Autodesk Fusion 360 part; units mm, degrees
(part 3 of 4)
sketch "Esboço7" plane through (0, 0, 2) normal (0, 0, 1) x (-1, 0, 0)
  arc A0 (-89.8492, -89.6213) -> (-86.4551, -92.1669) centre (-86.8794, -89.1971) ccw
  arc A1 (-79.6669, -98.9551) -> (-86.4551, -92.1669) centre (-85.6066, -98.1066) ccw
  arc A2 (-79.6669, -98.9551) -> (-77.1213, -102.3492) centre (-76.6971, -99.3794) ccw
  arc A3 (-77.1213, -102.3492) -> (-73.7447, -102.4474) centre (-75, -87.5) ccw
  arc A4 (-46.7294, -108.889) -> (-73.7447, -102.4474) centre (-70.0264, -146.7235) ccw
  arc A5 (72.6915, -102.3213) -> (44.7852, -108.3244) centre (66.5604, -141.6847) ccw
  arc A6 (72.6915, -102.3213) -> (77.1213, -102.3492) centre (75, -87.5) ccw
  arc A7 (77.1213, -102.3492) -> (79.6669, -98.9551) centre (76.6971, -99.3794) ccw
  arc A8 (86.4551, -92.1669) -> (79.6669, -98.9551) centre (85.6066, -98.1066) ccw
  arc A9 (86.4551, -92.1669) -> (89.8492, -89.6213) centre (86.8794, -89.1971) ccw
  arc A10 (89.8492, -89.6213) -> (89.8492, -85.3787) centre (75, -87.5) ccw
  arc A11 (89.8492, -85.3787) -> (86.4551, -82.8331) centre (86.8794, -85.8029) ccw
  arc A12 (79.7798, -75.4623) -> (86.4551, -82.8331) centre (85.6066, -76.8934) ccw
  arc A13 (79.7798, -75.4623) -> (78.5519, -72.265) centre (76.8663, -74.7468) ccw
  arc A14 (60.7593, -50.7677) -> (78.5519, -72.265) centre (106.6436, -30.9026) ccw
  line L0 (60.7593, -50.7677) -> (50.5773, -27.2494)
  arc A15 (51.0282, 29.3922) -> (50.5773, -27.2494) centre (114.8154, 0.5617) ccw
  line L1 (51.0282, 29.3922) -> (60.9948, 51.443)
  arc A16 (78.5458, 72.2669) -> (60.9948, 51.443) centre (106.557, 30.8499) ccw
  arc A17 (78.5458, 72.2669) -> (79.7789, 75.4657) centre (76.8651, 74.7519) ccw
  arc A18 (86.4551, 82.8331) -> (79.7789, 75.4657) centre (85.6066, 76.8934) ccw
  arc A19 (86.4551, 82.8331) -> (89.8492, 85.3787) centre (86.8794, 85.8029) ccw
  arc A20 (89.8492, 85.3787) -> (89.8492, 89.6213) centre (75, 87.5) ccw
  arc A21 (89.8492, 89.6213) -> (86.4551, 92.1669) centre (86.8794, 89.1971) ccw
  arc A22 (79.6669, 98.9551) -> (86.4551, 92.1669) centre (85.6066, 98.1066) ccw
  arc A23 (79.6669, 98.9551) -> (77.1213, 102.3492) centre (76.6971, 99.3794) ccw
  arc A24 (77.1213, 102.3492) -> (72.8787, 102.3492) centre (75, 87.5) ccw
  arc A25 (72.8787, 102.3492) -> (70.3331, 98.9551) centre (73.3029, 99.3794) ccw
  arc A26 (62.5456, 92.3982) -> (70.3331, 98.9551) centre (64.3934, 98.1066) ccw
  arc A27 (62.5456, 92.3982) -> (59.6541, 91.8087) centre (61.6216, 89.544) ccw
  arc A28 (44.4663, 82.7551) -> (59.6541, 91.8087) centre (26.8616, 129.5533) ccw
  arc A29 (-59.6538, 91.7779) -> (-44.9685, 82.7086) centre (-26.4329, 129.146) ccw
  arc A30 (-59.6538, 91.7779) -> (-62.5625, 92.3928) centre (-61.6471, 89.5359) ccw
  arc A31 (-70.3331, 98.9551) -> (-62.5625, 92.3928) centre (-64.3934, 98.1066) ccw
  arc A32 (-70.3331, 98.9551) -> (-72.8787, 102.3492) centre (-73.3029, 99.3794) ccw
  arc A33 (-72.8787, 102.3492) -> (-77.1213, 102.3492) centre (-75, 87.5) ccw
  arc A34 (-77.1213, 102.3492) -> (-79.6669, 98.9551) centre (-76.6971, 99.3794) ccw
  arc A35 (-86.4551, 92.1669) -> (-79.6669, 98.9551) centre (-85.6066, 98.1066) ccw
  arc A36 (-86.4551, 92.1669) -> (-89.8492, 89.6213) centre (-86.8794, 89.1971) ccw
  arc A37 (-89.8492, 89.6213) -> (-89.8492, 85.3787) centre (-75, 87.5) ccw
  arc A38 (-89.8492, 85.3787) -> (-86.4551, 82.8331) centre (-86.8794, 85.8029) ccw
  arc A39 (-79.7789, 75.4657) -> (-86.4551, 82.8331) centre (-85.6066, 76.8934) ccw
  arc A40 (-79.7789, 75.4657) -> (-78.5458, 72.2669) centre (-76.8651, 74.7519) ccw
  arc A41 (-60.9948, 51.443) -> (-78.5458, 72.2669) centre (-106.557, 30.8499) ccw
  line L2 (-60.9948, 51.443) -> (-51.0282, 29.3922)
  arc A42 (-50.5773, -27.2494) -> (-51.0282, 29.3922) centre (-114.8154, 0.5617) ccw
  line L3 (-50.5773, -27.2494) -> (-60.7593, -50.7677)
  arc A43 (-78.5519, -72.265) -> (-60.7593, -50.7677) centre (-106.6436, -30.9026) ccw
  arc A44 (-78.5519, -72.265) -> (-79.7798, -75.4623) centre (-76.8663, -74.7468) ccw
  arc A45 (-86.4551, -82.8331) -> (-79.7798, -75.4623) centre (-85.6066, -76.8934) ccw
  arc A46 (-86.4551, -82.8331) -> (-89.8492, -85.3787) centre (-86.8794, -85.8029) ccw
  arc A47 (-89.8492, -85.3787) -> (-89.8492, -89.6213) centre (-75, -87.5) ccw
  circle A48 centre (72.5, -95.6021) radius 1.5
  circle A49 centre (-83, -87.5005) radius 1.5
  circle A50 centre (-75.0002, 95.5) radius 1.5
  circle A51 centre (-67, 87.5002) radius 1.5
  circle A52 centre (83, 87.5) radius 1.5
  circle A53 centre (75, 79.5) radius 1.5
  circle A54 centre (-75, 87.5) radius 3
  circle A55 centre (-74.9995, -95.5) radius 1.5
  circle A56 centre (-75.0005, -79.5) radius 1.5
  circle A57 centre (64.5, -87.6021) radius 1.5
  circle A58 centre (80.5, -87.6021) radius 1.5
  circle A59 centre (-75, -87.5) radius 3
  circle A60 centre (-83, 87.4998) radius 1.5
  circle A61 centre (75, 95.5) radius 1.5
  circle A62 centre (75, 87.5) radius 3
  circle A63 centre (67, 87.5) radius 1.5
  circle A64 centre (-74.9998, 79.5) radius 1.5
  circle A65 centre (-67, -87.4995) radius 1.5
  circle A66 centre (75, -87.5) radius 3
  circle A67 centre (72.5, -79.6021) radius 1.5
  circle A68 centre (40.65, 50) radius 2.15
  arc A69 (-57.5607, 76.943) -> (-64.8173, 70.6939) centre (-60.2496, 72.7276) ccw
  line L4 (-57.5607, 76.943) -> (-49.4611, 71.7764)
  arc A70 (-47.15, 67.561) -> (-49.4611, 71.7764) centre (-52.15, 67.561) ccw
  line L5 (-47.15, 67.561) -> (-47.15, 42.4858)
  arc A71 (-47.4521, 41.7697) -> (-47.15, 42.4858) centre (-48.15, 42.4858) ccw
  line L6 (-47.4521, 41.7697) -> (-49.5538, 39.7214)
  arc A72 (-51.1653, 40.0309) -> (-49.5538, 39.7214) centre (-50.2517, 40.4376) ccw
  line L7 (-51.1653, 40.0309) -> (-64.8173, 70.6939)
  circle A73 centre (-40.65, 50) radius 2.15
  circle A74 centre (40.65, 60) radius 2.15
  line L8 (47.15, 42.4858) -> (47.15, 67.561)
  arc A75 (49.4611, 71.7764) -> (47.15, 67.561) centre (52.15, 67.561) ccw
  line L9 (49.4611, 71.7764) -> (57.5607, 76.943)
  arc A76 (64.8173, 70.6939) -> (57.5607, 76.943) centre (60.2496, 72.7276) ccw
  line L10 (64.8173, 70.6939) -> (51.1653, 40.0309)
  arc A77 (49.5538, 39.7214) -> (51.1653, 40.0309) centre (50.2517, 40.4376) ccw
  line L11 (49.5538, 39.7214) -> (47.4521, 41.7697)
  arc A78 (47.15, 42.4858) -> (47.4521, 41.7697) centre (48.15, 42.4858) ccw
  circle A79 centre (-40.65, 60) radius 2.15
  arc A80 (-10.473, -56.6595) -> (-14.3032, -58.4456) centre (-10.473, -61.6595) ccw
  line L12 (-10.473, -56.6595) -> (-7, -56.6595)
  arc A81 (-5, -58.6595) -> (-7, -56.6595) centre (-7, -58.6595) ccw
  line L13 (-5, -58.6595) -> (-5, -97.464)
  arc A82 (-9.1318, -102.3881) -> (-5, -97.464) centre (-10, -97.464) ccw
  line L14 (-9.1318, -102.3881) -> (-26.9725, -105.5339)
  arc A83 (-32.7648, -101.4781) -> (-26.9725, -105.5339) centre (-27.8408, -100.6098) ccw
  line L15 (-32.7648, -101.4781) -> (-35.4243, -86.3954)
  arc A84 (-34.3305, -82.3132) -> (-35.4243, -86.3954) centre (-30.5003, -85.5271) ccw
  line L16 (-34.3305, -82.3132) -> (-14.3032, -58.4456)
  arc A85 (-40.9054, 16.7074) -> (-37.3489, 15.6517) centre (-38.8619, 17.0732) ccw
  line L17 (-40.9054, 16.7074) -> (-46.7322, 29.5993)
  arc A86 (-44.339, 36.0244) -> (-46.7322, 29.5993) centre (-42.0339, 31.5075) ccw
  arc A87 (-44.339, 36.0244) -> (-34.6129, 45.4956) centre (-56.2565, 57.9923) ccw
  arc A88 (-28.1234, 47.5076) -> (-34.6129, 45.4956) centre (-30.28, 42.9921) ccw
  line L18 (-28.1234, 47.5076) -> (-14.9942, 41.2515)
  arc A89 (-14.46, 38.0146) -> (-14.9942, 41.2515) centre (-15.8549, 39.4469) ccw
  line L19 (-14.46, 38.0146) -> (-37.3489, 15.6517)
  line L20 (5, -97.464) -> (5, -58.6595)
  arc A90 (7, -56.6595) -> (5, -58.6595) centre (7, -58.6595) ccw
  line L21 (7, -56.6595) -> (10.473, -56.6595)
  arc A91 (14.3032, -58.4456) -> (10.473, -56.6595) centre (10.473, -61.6595) ccw
  line L22 (14.3032, -58.4456) -> (34.3305, -82.3132)
  arc A92 (35.4243, -86.3954) -> (34.3305, -82.3132) centre (30.5003, -85.5271) ccw
  line L23 (35.4243, -86.3954) -> (32.7648, -101.4781)
  arc A93 (26.9725, -105.5339) -> (32.7648, -101.4781) centre (27.8408, -100.6098) ccw
  line L24 (26.9725, -105.5339) -> (9.1318, -102.3881)
  arc A94 (5, -97.464) -> (9.1318, -102.3881) centre (10, -97.464) ccw
  arc A95 (-61.9967, -63.6938) -> (-55.4143, -68.0759) centre (-58.3695, -65.3802) ccw
  line L25 (-61.9967, -63.6938) -> (-41.8922, -17.2564)
  arc A96 (-36.246, -16.5772) -> (-41.8922, -17.2564) centre (-38.8636, -18.6251) ccw
  line L26 (-36.246, -16.5772) -> (-23.6374, -29.1331)
  arc A97 (-23.5625, -33.2372) -> (-23.6374, -29.1331) centre (-25.7596, -31.2246) ccw
  line L27 (-23.5625, -33.2372) -> (-55.4143, -68.0759)
  arc A98 (38.1376, -9.2791) -> (38.7256, -7.6527) centre (36.7356, -7.8528) ccw
  line L28 (38.1376, -9.2791) -> (27.9736, -19.2699)
  arc A99 (24.5716, -17.8424) -> (27.9736, -19.2699) centre (26.5716, -17.8436) ccw
  line L29 (24.5716, -17.8424) -> (24.5916, 17.8264)
  arc A100 (27.9955, 19.2498) -> (24.5916, 17.8264) centre (26.5916, 17.8253) ccw
  line L30 (27.9955, 19.2498) -> (38.1463, 9.2454)
  arc A101 (38.7321, 7.6192) -> (38.1463, 9.2454) centre (36.7424, 7.821) ccw
  arc A102 (38.7321, 7.6192) -> (38.7256, -7.6527) centre (114.3432, -0.0492) ccw
  arc A103 (9.266, 38.142) -> (7.6383, 38.7303) centre (7.8393, 36.7404) ccw
  line L31 (9.266, 38.142) -> (19.2664, 27.9622)
  arc A104 (17.8415, 24.5606) -> (19.2664, 27.9622) centre (17.8397, 26.5606) ccw
  line L32 (17.8415, 24.5606) -> (-17.871, 24.5283)
  arc A105 (-19.3052, 27.9241) -> (-17.871, 24.5283) centre (-17.8728, 26.5283) ccw
  line L33 (-19.3052, 27.9241) -> (-9.3455, 38.1438)
  arc A106 (-7.7103, 38.7376) -> (-9.3455, 38.1438) centre (-7.9132, 36.7479) ccw
  arc A107 (-7.7103, 38.7376) -> (7.6383, 38.7303) centre (0, 114.3455) ccw
  line L34 (41.7895, -17.0192) -> (61.9965, -63.6935)
  arc A108 (55.3948, -68.0303) -> (61.9965, -63.6935) centre (58.3475, -65.3318) ccw
  line L35 (55.3948, -68.0303) -> (23.5953, -33.2362)
  arc A109 (23.7067, -29.0729) -> (23.5953, -33.2362) centre (25.8097, -31.2123) ccw
  line L36 (23.7067, -29.0729) -> (36.9334, -16.0716)
  arc A110 (41.7895, -17.0192) -> (36.9334, -16.0716) centre (39.0364, -18.2111) ccw
  arc A111 (37.4337, 15.5639) -> (40.6601, 16.1647) centre (38.8376, 16.9884) ccw
  line L37 (37.4337, 15.5639) -> (14.6425, 38.0264)
  arc A112 (15.1963, 41.2612) -> (14.6425, 38.0264) centre (16.0464, 39.4508) ccw
  line L38 (15.1963, 41.2612) -> (28.3187, 47.4234)
  arc A113 (34.7856, 45.3775) -> (28.3187, 47.4234) centre (30.444, 42.8975) ccw
  arc A114 (34.7856, 45.3775) -> (44.4886, 35.8486) centre (56.4937, 57.7776) ccw
  arc A115 (46.6438, 29.4035) -> (44.4886, 35.8486) centre (42.0875, 31.4628) ccw
  line L39 (46.6438, 29.4035) -> (40.6601, 16.1647)
  line L40 (19.3052, -27.9241) -> (9.3455, -38.1438)
  arc A116 (7.7103, -38.7376) -> (9.3455, -38.1438) centre (7.9132, -36.7479) ccw
  arc A117 (7.7103, -38.7376) -> (-7.6383, -38.7303) centre (0, -114.3455) ccw
  arc A118 (-9.266, -38.142) -> (-7.6383, -38.7303) centre (-7.8393, -36.7404) ccw
  line L41 (-9.266, -38.142) -> (-19.2664, -27.9622)
  arc A119 (-17.8415, -24.5606) -> (-19.2664, -27.9622) centre (-17.8397, -26.5606) ccw
  line L42 (-17.8415, -24.5606) -> (17.871, -24.5283)
  arc A120 (19.3052, -27.9241) -> (17.871, -24.5283) centre (17.8728, -26.5283) ccw
  arc A121 (-38.7303, -7.6383) -> (-38.142, -9.266) centre (-36.7404, -7.8393) ccw
  arc A122 (-38.7303, -7.6383) -> (-38.7376, 7.7103) centre (-114.3455, 0) ccw
  arc A123 (-38.1438, 9.3455) -> (-38.7376, 7.7103) centre (-36.7479, 7.9132) ccw
  line L43 (-38.1438, 9.3455) -> (-27.9241, 19.3052)
  arc A124 (-24.5283, 17.871) -> (-27.9241, 19.3052) centre (-26.5283, 17.8728) ccw
  line L44 (-24.5283, 17.871) -> (-24.5606, -17.8415)
  arc A125 (-27.9622, -19.2664) -> (-24.5607, -17.8415) centre (-26.5606, -17.8397) ccw
  line L45 (-27.9622, -19.2664) -> (-38.142, -9.266)
  circle A126 centre (-10.25, -46.6) radius 1.5
  line L46 (8, -42.5) -> (8, -50.7)
  line L47 (8, -50.7) -> (-8, -50.7)
  line L48 (-8, -50.7) -> (-8, -42.5)
  line L49 (-8, -42.5) -> (8, -42.5)
  circle A127 centre (10.25, -46.6) radius 1.5
  circle A128 centre (-50, 0) radius 2.15
  arc A129 (-50.5733, 28.3637) -> (-50.5773, -27.2494) centre (35.4576, 0.5509) ccw
  line L50 (0, 0) -> (0, -46.9846) construction
  circle A130 centre (50, 0) radius 2.15
  arc A131 (50.5773, -27.2494) -> (50.5733, 28.3637) centre (-35.4576, 0.5509) ccw
  line L51 (35.9657, 79.8952) -> (2.1827, 93.0889)
  arc A132 (2.1827, 93.0889) -> (-2.1423, 93.1045) centre (0, 87.5) ccw
  line L52 (0, 81.5) -> (15.6612, 75.3836)
  line L53 (-16.4256, 75.2214) -> (0, 81.5)
  line L54 (-2.1423, 93.1045) -> (-36.9275, 79.8081)
  arc A133 (6.7322, 8.1464) -> (6.3787, 9) centre (6.3787, 8.5) ccw
  line L55 (6.7322, 8.1464) -> (0.7071, 2.1213)
  arc A134 (-0.7071, 2.1213) -> (0.7071, 2.1213) centre (0, 2.8284) ccw
  line L56 (-0.7071, 2.1213) -> (-6.7322, 8.1464)
  arc A135 (-6.3787, 9) -> (-6.7322, 8.1464) centre (-6.3787, 8.5) ccw
  line L57 (-6.3787, 9) -> (6.3787, 9)
  arc A136 (-8.1464, 6.7322) -> (-9, 6.3787) centre (-8.5, 6.3787) ccw
  line L58 (-8.1464, 6.7322) -> (-2.1213, 0.7071)
  arc A137 (-2.1213, -0.7071) -> (-2.1213, 0.7071) centre (-2.8284, 0) ccw
  line L59 (-2.1213, -0.7071) -> (-8.1464, -6.7322)
  arc A138 (-9, -6.3787) -> (-8.1464, -6.7322) centre (-8.5, -6.3787) ccw
  line L60 (-9, -6.3787) -> (-9, 6.3787)
  arc A139 (-6.7322, -8.1464) -> (-6.3787, -9) centre (-6.3787, -8.5) ccw
  line L61 (-6.7322, -8.1464) -> (-0.7071, -2.1213)
  arc A140 (0.7071, -2.1213) -> (-0.7071, -2.1213) centre (0, -2.8284) ccw
  line L62 (0.7071, -2.1213) -> (6.7322, -8.1464)
  arc A141 (6.3787, -9) -> (6.7322, -8.1464) centre (6.3787, -8.5) ccw
  line L63 (6.3787, -9) -> (-6.3787, -9)
  line L64 (8.1464, -6.7322) -> (2.1213, -0.7071)
  arc A142 (2.1213, 0.7071) -> (2.1213, -0.7071) centre (2.8284, 0) ccw
  line L65 (2.1213, 0.7071) -> (8.1464, 6.7322)
  arc A143 (9, 6.3787) -> (8.1464, 6.7322) centre (8.5, 6.3787) ccw
  line L66 (9, 6.3787) -> (9, -6.3787)
  arc A144 (8.1464, -6.7322) -> (9, -6.3787) centre (8.5, -6.3787) ccw
  circle A145 centre (0, 87.5) radius 2.15
  arc A146 (26.2105, 50.915) -> (27.5676, 55.0697) centre (24.9353, 53.6305) ccw
  line L67 (26.2105, 50.915) -> (10.6059, 43.5872)
  arc A147 (9.3307, 43.3027) -> (10.6059, 43.5872) centre (9.3307, 46.3027) ccw
  line L68 (9.3307, 43.3027) -> (-9.3218, 43.3027)
  arc A148 (-10.6123, 43.5944) -> (-9.3218, 43.3027) centre (-9.3218, 46.3027) ccw
  line L69 (-10.6123, 43.5944) -> (-26.8632, 51.3381)
  arc A149 (-28.1945, 55.5044) -> (-26.8632, 51.3381) centre (-25.5727, 54.0463) ccw
  line L70 (-28.1945, 55.5044) -> (-17.9762, 73.8773)
  arc A150 (-16.4256, 75.2214) -> (-17.9762, 73.8773) centre (-15.3544, 72.4192) ccw
  arc A151 (17.2021, 74.0283) -> (15.6612, 75.3836) centre (14.5698, 72.5892) ccw
  line L71 (17.2021, 74.0283) -> (27.5676, 55.0697)
  arc A152 (-46.7294, -108.889) -> (-25.7561, -114.8285) centre (-25.7561, -74.8285) ccw
  line L72 (-25.7561, -114.8285) -> (22.9214, -114.8285)
  arc A153 (22.9214, -114.8285) -> (44.7852, -108.3244) centre (22.9214, -74.8285) ccw
  circle A154 centre (-10, 10) radius 3
  circle A155 centre (10, -10) radius 3
  circle A156 centre (-10, -10) radius 3
  circle A157 centre (10, 10) radius 3
  arc A158 (35.9657, 79.8952) -> (44.4663, 82.7551) centre (-0.31, 201.7835) ccw
  arc A159 (-44.9685, 82.7086) -> (-36.9275, 79.8081) centre (2.2046, 200.8918) ccw
  point P0 (-72.5, 87.3979)
  point P1 (-72.5, -87.6021)
  point P2 (72.5, 87.3979)
  point P3 (72.5, -87.6021)
  point P4 (-72.5, 87.3979)
  point P5 (-72.5, -87.6021)
  point P6 (72.5, 87.3979)
  point P7 (72.5, -87.6021)
  point P8 (-72.5, 87.3979)
  point P9 (-72.5, -87.6021)
  point P10 (72.5, 87.3979)
  point P11 (72.5, -87.6021)
  point P12 (-72.5, 87.3979)
  point P13 (-72.5, -87.6021)
  point P14 (72.5, 87.3979)
  point P15 (72.5, -87.6021)
  point P16 (-72.5, 87.3979)
  point P17 (-72.5, -87.6021)
  point P18 (72.5, 87.3979)
  point P19 (72.5, -87.6021)
  point P20 (72.5, -87.6021)
  point P21 (72.5, -87.6021)
  point P22 (72.5, -87.6021)
  point P23 (72.5, -87.6021)
  dimension "d142" = 4.3
  dimension "d143" = 50
  dimension "d144" = 90.4149
  constraint coincident A42.start L3.start
  constraint coincident L50.start origin
  constraint perpendicular L49 L50
  constraint symmetric A128 L50 A130
  constraint symmetric A42.start L50 L0.end
  constraint symmetric A129.start L50 A131.end
  constraint symmetric A129 L50 A131
  constraint coincident A15 A131.end
  measures "d142" diameter of A128
  measures "d143" distance of L50.start A128.centre
  measures "d144" radius of A129
extrude "Extrusão9" add sketch "Esboço7" against normal blind 4 contours A42 A129 | A15 A131
fillet "Arredondamento3" radius 15 4 edges at (50.5733, -28.3637, 0) (50.5773, 27.2494, 0) (-50.5733, -28.3637, 0) (-50.5773, 27.2494, 0)
sketch "Esboço8" plane through (0, 0, 2) normal (0, 0, 1) x (-1, 0, 0)
  circle A0 centre (-50, 0) radius 2.15
  circle A1 centre (50, 0) radius 2.15
  arc A2 (-89.8492, -89.6213) -> (-86.4551, -92.1669) centre (-86.8794, -89.1971) ccw
  arc A3 (-79.6669, -98.9551) -> (-86.4551, -92.1669) centre (-85.6066, -98.1066) ccw
  arc A4 (-79.6669, -98.9551) -> (-77.1213, -102.3492) centre (-76.6971, -99.3794) ccw
  arc A5 (-77.1213, -102.3492) -> (-73.7447, -102.4474) centre (-75, -87.5) ccw
  arc A6 (-46.7294, -108.889) -> (-73.7447, -102.4474) centre (-70.0264, -146.7235) ccw
  arc A7 (72.6915, -102.3213) -> (44.7852, -108.3244) centre (66.5604, -141.6847) ccw
  arc A8 (72.6915, -102.3213) -> (77.1213, -102.3492) centre (75, -87.5) ccw
  arc A9 (77.1213, -102.3492) -> (79.6669, -98.9551) centre (76.6971, -99.3794) ccw
  arc A10 (86.4551, -92.1669) -> (79.6669, -98.9551) centre (85.6066, -98.1066) ccw
  arc A11 (86.4551, -92.1669) -> (89.8492, -89.6213) centre (86.8794, -89.1971) ccw
  arc A12 (89.8492, -89.6213) -> (89.8492, -85.3787) centre (75, -87.5) ccw
  arc A13 (89.8492, -85.3787) -> (86.4551, -82.8331) centre (86.8794, -85.8029) ccw
  arc A14 (79.7798, -75.4623) -> (86.4551, -82.8331) centre (85.6066, -76.8934) ccw
  arc A15 (79.7798, -75.4623) -> (78.5519, -72.265) centre (76.8663, -74.7468) ccw
  arc A16 (60.7593, -50.7677) -> (78.5519, -72.265) centre (106.6436, -30.9026) ccw
  line L0 (60.7593, -50.7677) -> (52.7268, -32.2145)
  arc A17 (51.9852, -22.4406) -> (52.7268, -32.2145) centre (66.4922, -26.2549) ccw
  arc A18 (51.9852, -22.4406) -> (52.0095, 23.4499) centre (-35.4576, 0.5509) ccw
  arc A19 (52.8518, 33.4268) -> (52.0095, 23.4499) centre (66.5205, 27.2489) ccw
  line L1 (52.8518, 33.4268) -> (60.9948, 51.443)
  arc A20 (78.5458, 72.2669) -> (60.9948, 51.443) centre (106.557, 30.8499) ccw
  arc A21 (78.5458, 72.2669) -> (79.7789, 75.4657) centre (76.8651, 74.7519) ccw
  arc A22 (86.4551, 82.8331) -> (79.7789, 75.4657) centre (85.6066, 76.8934) ccw
  arc A23 (86.4551, 82.8331) -> (89.8492, 85.3787) centre (86.8794, 85.8029) ccw
  arc A24 (89.8492, 85.3787) -> (89.8492, 89.6213) centre (75, 87.5) ccw
  arc A25 (89.8492, 89.6213) -> (86.4551, 92.1669) centre (86.8794, 89.1971) ccw
  arc A26 (79.6669, 98.9551) -> (86.4551, 92.1669) centre (85.6066, 98.1066) ccw
  arc A27 (79.6669, 98.9551) -> (77.1213, 102.3492) centre (76.6971, 99.3794) ccw
  arc A28 (77.1213, 102.3492) -> (72.8787, 102.3492) centre (75, 87.5) ccw
  arc A29 (72.8787, 102.3492) -> (70.3331, 98.9551) centre (73.3029, 99.3794) ccw
  arc A30 (62.5456, 92.3982) -> (70.3331, 98.9551) centre (64.3934, 98.1066) ccw
  arc A31 (62.5456, 92.3982) -> (59.6541, 91.8087) centre (61.6216, 89.544) ccw
  arc A32 (44.4663, 82.7551) -> (59.6541, 91.8087) centre (26.8616, 129.5533) ccw
  arc A33 (-59.6538, 91.7779) -> (-44.9685, 82.7086) centre (-26.4329, 129.146) ccw
  arc A34 (-59.6538, 91.7779) -> (-62.5625, 92.3928) centre (-61.6471, 89.5359) ccw
  arc A35 (-70.3331, 98.9551) -> (-62.5625, 92.3928) centre (-64.3934, 98.1066) ccw
  arc A36 (-70.3331, 98.9551) -> (-72.8787, 102.3492) centre (-73.3029, 99.3794) ccw
  arc A37 (-72.8787, 102.3492) -> (-77.1213, 102.3492) centre (-75, 87.5) ccw
  arc A38 (-77.1213, 102.3492) -> (-79.6669, 98.9551) centre (-76.6971, 99.3794) ccw
  arc A39 (-86.4551, 92.1669) -> (-79.6669, 98.9551) centre (-85.6066, 98.1066) ccw
  arc A40 (-86.4551, 92.1669) -> (-89.8492, 89.6213) centre (-86.8794, 89.1971) ccw
  arc A41 (-89.8492, 89.6213) -> (-89.8492, 85.3787) centre (-75, 87.5) ccw
  arc A42 (-89.8492, 85.3787) -> (-86.4551, 82.8331) centre (-86.8794, 85.8029) ccw
  arc A43 (-79.7789, 75.4657) -> (-86.4551, 82.8331) centre (-85.6066, 76.8934) ccw
  arc A44 (-79.7789, 75.4657) -> (-78.5458, 72.2669) centre (-76.8651, 74.7519) ccw
  arc A45 (-60.9948, 51.443) -> (-78.5458, 72.2669) centre (-106.557, 30.8499) ccw
  line L2 (-60.9948, 51.443) -> (-52.8518, 33.4268)
  arc A46 (-52.0095, 23.4499) -> (-52.8518, 33.4268) centre (-66.5205, 27.2489) ccw
  arc A47 (-52.0095, 23.4499) -> (-51.9852, -22.4406) centre (35.4576, 0.5509) ccw
  arc A48 (-52.7268, -32.2145) -> (-51.9852, -22.4406) centre (-66.4922, -26.2549) ccw
  line L3 (-52.7268, -32.2145) -> (-60.7593, -50.7677)
  arc A49 (-78.5519, -72.265) -> (-60.7593, -50.7677) centre (-106.6436, -30.9026) ccw
  arc A50 (-78.5519, -72.265) -> (-79.7798, -75.4623) centre (-76.8663, -74.7468) ccw
  arc A51 (-86.4551, -82.8331) -> (-79.7798, -75.4623) centre (-85.6066, -76.8934) ccw
  arc A52 (-86.4551, -82.8331) -> (-89.8492, -85.3787) centre (-86.8794, -85.8029) ccw
  arc A53 (-89.8492, -85.3787) -> (-89.8492, -89.6213) centre (-75, -87.5) ccw
  circle A54 centre (72.5, -95.6021) radius 1.5
  circle A55 centre (-83, -87.5005) radius 1.5
  circle A56 centre (-75.0002, 95.5) radius 1.5
  circle A57 centre (-67, 87.5002) radius 1.5
  circle A58 centre (83, 87.5) radius 1.5
  circle A59 centre (75, 79.5) radius 1.5
  circle A60 centre (-75, 87.5) radius 3
  circle A61 centre (-74.9995, -95.5) radius 1.5
  circle A62 centre (-75.0005, -79.5) radius 1.5
  circle A63 centre (64.5, -87.6021) radius 1.5
  circle A64 centre (80.5, -87.6021) radius 1.5
  circle A65 centre (-75, -87.5) radius 3
  circle A66 centre (-83, 87.4998) radius 1.5
  circle A67 centre (75, 95.5) radius 1.5
  circle A68 centre (75, 87.5) radius 3
  circle A69 centre (67, 87.5) radius 1.5
  circle A70 centre (-74.9998, 79.5) radius 1.5
  circle A71 centre (-67, -87.4995) radius 1.5
  circle A72 centre (75, -87.5) radius 3
  circle A73 centre (72.5, -79.6021) radius 1.5
  circle A74 centre (40.65, 50) radius 2.15
  arc A75 (-57.5607, 76.943) -> (-64.8173, 70.6939) centre (-60.2496, 72.7276) ccw
  line L4 (-57.5607, 76.943) -> (-49.4611, 71.7764)
  arc A76 (-47.15, 67.561) -> (-49.4611, 71.7764) centre (-52.15, 67.561) ccw
  line L5 (-47.15, 67.561) -> (-47.15, 42.4858)
  arc A77 (-47.4521, 41.7697) -> (-47.15, 42.4858) centre (-48.15, 42.4858) ccw
  line L6 (-47.4521, 41.7697) -> (-49.5538, 39.7214)
  arc A78 (-51.1653, 40.0309) -> (-49.5538, 39.7214) centre (-50.2517, 40.4376) ccw
  line L7 (-51.1653, 40.0309) -> (-64.8173, 70.6939)
  circle A79 centre (-40.65, 50) radius 2.15
  circle A80 centre (40.65, 60) radius 2.15
  line L8 (47.15, 42.4858) -> (47.15, 67.561)
  arc A81 (49.4611, 71.7764) -> (47.15, 67.561) centre (52.15, 67.561) ccw
  line L9 (49.4611, 71.7764) -> (57.5607, 76.943)
  arc A82 (64.8173, 70.6939) -> (57.5607, 76.943) centre (60.2496, 72.7276) ccw
  line L10 (64.8173, 70.6939) -> (51.1653, 40.0309)
  arc A83 (49.5538, 39.7214) -> (51.1653, 40.0309) centre (50.2517, 40.4376) ccw
  line L11 (49.5538, 39.7214) -> (47.4521, 41.7697)
  arc A84 (47.15, 42.4858) -> (47.4521, 41.7697) centre (48.15, 42.4858) ccw
  circle A85 centre (-40.65, 60) radius 2.15
  arc A86 (-10.473, -56.6595) -> (-14.3032, -58.4456) centre (-10.473, -61.6595) ccw
  line L12 (-10.473, -56.6595) -> (-7, -56.6595)
  arc A87 (-5, -58.6595) -> (-7, -56.6595) centre (-7, -58.6595) ccw
  line L13 (-5, -58.6595) -> (-5, -97.464)
  arc A88 (-9.1318, -102.3881) -> (-5, -97.464) centre (-10, -97.464) ccw
  line L14 (-9.1318, -102.3881) -> (-26.9725, -105.5339)
  arc A89 (-32.7648, -101.4781) -> (-26.9725, -105.5339) centre (-27.8408, -100.6098) ccw
  line L15 (-32.7648, -101.4781) -> (-35.4243, -86.3954)
  arc A90 (-34.3305, -82.3132) -> (-35.4243, -86.3954) centre (-30.5003, -85.5271) ccw
  line L16 (-34.3305, -82.3132) -> (-14.3032, -58.4456)
  arc A91 (-40.9054, 16.7074) -> (-37.3489, 15.6517) centre (-38.8619, 17.0732) ccw
  line L17 (-40.9054, 16.7074) -> (-46.7322, 29.5993)
  arc A92 (-44.339, 36.0244) -> (-46.7322, 29.5993) centre (-42.0339, 31.5075) ccw
  arc A93 (-44.339, 36.0244) -> (-34.6129, 45.4956) centre (-56.2565, 57.9923) ccw
  arc A94 (-28.1234, 47.5076) -> (-34.6129, 45.4956) centre (-30.28, 42.9921) ccw
  line L18 (-28.1234, 47.5076) -> (-14.9942, 41.2515)
  arc A95 (-14.46, 38.0146) -> (-14.9942, 41.2515) centre (-15.8549, 39.4469) ccw
  line L19 (-14.46, 38.0146) -> (-37.3489, 15.6517)
  line L20 (5, -97.464) -> (5, -58.6595)
  arc A96 (7, -56.6595) -> (5, -58.6595) centre (7, -58.6595) ccw
  line L21 (7, -56.6595) -> (10.473, -56.6595)
  arc A97 (14.3032, -58.4456) -> (10.473, -56.6595) centre (10.473, -61.6595) ccw
  line L22 (14.3032, -58.4456) -> (34.3305, -82.3132)
  arc A98 (35.4243, -86.3954) -> (34.3305, -82.3132) centre (30.5003, -85.5271) ccw
  line L23 (35.4243, -86.3954) -> (32.7648, -101.4781)
  arc A99 (26.9725, -105.5339) -> (32.7648, -101.4781) centre (27.8408, -100.6098) ccw
  line L24 (26.9725, -105.5339) -> (9.1318, -102.3881)
  arc A100 (5, -97.464) -> (9.1318, -102.3881) centre (10, -97.464) ccw
  arc A101 (-61.9967, -63.6938) -> (-55.4143, -68.0759) centre (-58.3695, -65.3802) ccw
  line L25 (-61.9967, -63.6938) -> (-41.8922, -17.2564)
  arc A102 (-36.246, -16.5772) -> (-41.8922, -17.2564) centre (-38.8636, -18.6251) ccw
  line L26 (-36.246, -16.5772) -> (-23.6374, -29.1331)
  arc A103 (-23.5625, -33.2372) -> (-23.6374, -29.1331) centre (-25.7596, -31.2246) ccw
  line L27 (-23.5625, -33.2372) -> (-55.4143, -68.0759)
  arc A104 (38.1376, -9.2791) -> (38.7256, -7.6527) centre (36.7356, -7.8528) ccw
  line L28 (38.1376, -9.2791) -> (27.9736, -19.2699)
  arc A105 (24.5716, -17.8424) -> (27.9736, -19.2699) centre (26.5716, -17.8436) ccw
  line L29 (24.5716, -17.8424) -> (24.5916, 17.8264)
  arc A106 (27.9955, 19.2498) -> (24.5916, 17.8264) centre (26.5916, 17.8253) ccw
  line L30 (27.9955, 19.2498) -> (38.1463, 9.2454)
  arc A107 (38.7321, 7.6192) -> (38.1463, 9.2454) centre (36.7424, 7.821) ccw
  arc A108 (38.7321, 7.6192) -> (38.7256, -7.6527) centre (114.3432, -0.0492) ccw
  arc A109 (9.266, 38.142) -> (7.6383, 38.7303) centre (7.8393, 36.7404) ccw
  line L31 (9.266, 38.142) -> (19.2664, 27.9622)
  arc A110 (17.8415, 24.5606) -> (19.2664, 27.9622) centre (17.8397, 26.5606) ccw
  line L32 (17.8415, 24.5606) -> (-17.871, 24.5283)
  arc A111 (-19.3052, 27.9241) -> (-17.871, 24.5283) centre (-17.8728, 26.5283) ccw
  line L33 (-19.3052, 27.9241) -> (-9.3455, 38.1438)
  arc A112 (-7.7103, 38.7376) -> (-9.3455, 38.1438) centre (-7.9132, 36.7479) ccw
  arc A113 (-7.7103, 38.7376) -> (7.6383, 38.7303) centre (0, 114.3455) ccw
  line L34 (41.7895, -17.0192) -> (61.9965, -63.6935)
  arc A114 (55.3948, -68.0303) -> (61.9965, -63.6935) centre (58.3475, -65.3318) ccw
  line L35 (55.3948, -68.0303) -> (23.5953, -33.2362)
  arc A115 (23.7067, -29.0729) -> (23.5953, -33.2362) centre (25.8097, -31.2123) ccw
  line L36 (23.7067, -29.0729) -> (36.9334, -16.0716)
  arc A116 (41.7895, -17.0192) -> (36.9334, -16.0716) centre (39.0364, -18.2111) ccw
  arc A117 (37.4337, 15.5639) -> (40.6601, 16.1647) centre (38.8376, 16.9884) ccw
  line L37 (37.4337, 15.5639) -> (14.6425, 38.0264)
  arc A118 (15.1963, 41.2612) -> (14.6425, 38.0264) centre (16.0464, 39.4508) ccw
  line L38 (15.1963, 41.2612) -> (28.3187, 47.4234)
  arc A119 (34.7856, 45.3775) -> (28.3187, 47.4234) centre (30.444, 42.8975) ccw
  arc A120 (34.7856, 45.3775) -> (44.4886, 35.8486) centre (56.4937, 57.7776) ccw
  arc A121 (46.6438, 29.4035) -> (44.4886, 35.8486) centre (42.0875, 31.4628) ccw
  line L39 (46.6438, 29.4035) -> (40.6601, 16.1647)
  line L40 (19.3052, -27.9241) -> (9.3455, -38.1438)
  arc A122 (7.7103, -38.7376) -> (9.3455, -38.1438) centre (7.9132, -36.7479) ccw
  arc A123 (7.7103, -38.7376) -> (-7.6383, -38.7303) centre (0, -114.3455) ccw
  arc A124 (-9.266, -38.142) -> (-7.6383, -38.7303) centre (-7.8393, -36.7404) ccw
  line L41 (-9.266, -38.142) -> (-19.2664, -27.9622)
  arc A125 (-17.8415, -24.5606) -> (-19.2664, -27.9622) centre (-17.8397, -26.5606) ccw
  line L42 (-17.8415, -24.5606) -> (17.871, -24.5283)
  arc A126 (19.3052, -27.9241) -> (17.871, -24.5283) centre (17.8728, -26.5283) ccw
  arc A127 (-38.7303, -7.6383) -> (-38.142, -9.266) centre (-36.7404, -7.8393) ccw
  arc A128 (-38.7303, -7.6383) -> (-38.7376, 7.7103) centre (-114.3455, 0) ccw
  arc A129 (-38.1438, 9.3455) -> (-38.7376, 7.7103) centre (-36.7479, 7.9132) ccw
  line L43 (-38.1438, 9.3455) -> (-27.9241, 19.3052)
  arc A130 (-24.5283, 17.871) -> (-27.9241, 19.3052) centre (-26.5283, 17.8728) ccw
  line L44 (-24.5283, 17.871) -> (-24.5606, -17.8415)
  arc A131 (-27.9622, -19.2664) -> (-24.5607, -17.8415) centre (-26.5606, -17.8397) ccw
  line L45 (-27.9622, -19.2664) -> (-38.142, -9.266)
  circle A132 centre (-10.25, -46.6) radius 1.5
  line L46 (8, -42.5) -> (8, -50.7)
  line L47 (8, -50.7) -> (-8, -50.7)
  line L48 (-8, -50.7) -> (-8, -42.5)
  line L49 (-8, -42.5) -> (8, -42.5)
  circle A133 centre (10.25, -46.6) radius 1.5
  line L50 (35.9657, 79.8952) -> (2.1827, 93.0889)
  arc A134 (2.1827, 93.0889) -> (-2.1423, 93.1045) centre (0, 87.5) ccw
  line L51 (0, 81.5) -> (15.6612, 75.3836)
  line L52 (-16.4256, 75.2214) -> (0, 81.5)
  line L53 (-2.1423, 93.1045) -> (-36.9275, 79.8081)
  arc A135 (6.7322, 8.1464) -> (6.3787, 9) centre (6.3787, 8.5) ccw
  line L54 (6.7322, 8.1464) -> (0.7071, 2.1213)
  arc A136 (-0.7071, 2.1213) -> (0.7071, 2.1213) centre (0, 2.8284) ccw
  line L55 (-0.7071, 2.1213) -> (-6.7322, 8.1464)
  arc A137 (-6.3787, 9) -> (-6.7322, 8.1464) centre (-6.3787, 8.5) ccw
  line L56 (-6.3787, 9) -> (6.3787, 9)
  arc A138 (-8.1464, 6.7322) -> (-9, 6.3787) centre (-8.5, 6.3787) ccw
  line L57 (-8.1464, 6.7322) -> (-2.1213, 0.7071)
  arc A139 (-2.1213, -0.7071) -> (-2.1213, 0.7071) centre (-2.8284, 0) ccw
  line L58 (-2.1213, -0.7071) -> (-8.1464, -6.7322)
  arc A140 (-9, -6.3787) -> (-8.1464, -6.7322) centre (-8.5, -6.3787) ccw
  line L59 (-9, -6.3787) -> (-9, 6.3787)
  arc A141 (-6.7322, -8.1464) -> (-6.3787, -9) centre (-6.3787, -8.5) ccw
  line L60 (-6.7322, -8.1464) -> (-0.7071, -2.1213)
  arc A142 (0.7071, -2.1213) -> (-0.7071, -2.1213) centre (0, -2.8284) ccw
  line L61 (0.7071, -2.1213) -> (6.7322, -8.1464)
  arc A143 (6.3787, -9) -> (6.7322, -8.1464) centre (6.3787, -8.5) ccw
  line L62 (6.3787, -9) -> (-6.3787, -9)
  line L63 (8.1464, -6.7322) -> (2.1213, -0.7071)
  arc A144 (2.1213, 0.7071) -> (2.1213, -0.7071) centre (2.8284, 0) ccw
  line L64 (2.1213, 0.7071) -> (8.1464, 6.7322)
  arc A145 (9, 6.3787) -> (8.1464, 6.7322) centre (8.5, 6.3787) ccw
  line L65 (9, 6.3787) -> (9, -6.3787)
  arc A146 (8.1464, -6.7322) -> (9, -6.3787) centre (8.5, -6.3787) ccw
  circle A147 centre (0, 87.5) radius 2.15
  arc A148 (26.2105, 50.915) -> (27.5676, 55.0697) centre (24.9353, 53.6305) ccw
  line L66 (26.2105, 50.915) -> (10.6059, 43.5872)
  arc A149 (9.3307, 43.3027) -> (10.6059, 43.5872) centre (9.3307, 46.3027) ccw
  line L67 (9.3307, 43.3027) -> (-9.3218, 43.3027)
  arc A150 (-10.6123, 43.5944) -> (-9.3218, 43.3027) centre (-9.3218, 46.3027) ccw
  line L68 (-10.6123, 43.5944) -> (-26.8632, 51.3381)
  arc A151 (-28.1945, 55.5044) -> (-26.8632, 51.3381) centre (-25.5727, 54.0463) ccw
  line L69 (-28.1945, 55.5044) -> (-17.9762, 73.8773)
  arc A152 (-16.4256, 75.2214) -> (-17.9762, 73.8773) centre (-15.3544, 72.4192) ccw
  arc A153 (17.2021, 74.0283) -> (15.6612, 75.3836) centre (14.5698, 72.5892) ccw
  line L70 (17.2021, 74.0283) -> (27.5676, 55.0697)
  arc A154 (-46.7294, -108.889) -> (-25.7561, -114.8285) centre (-25.7561, -74.8285) ccw
  line L71 (-25.7561, -114.8285) -> (22.9214, -114.8285)
  arc A155 (22.9214, -114.8285) -> (44.7852, -108.3244) centre (22.9214, -74.8285) ccw
  circle A156 centre (-10, 10) radius 3
  circle A157 centre (10, -10) radius 3
  circle A158 centre (-10, -10) radius 3
  circle A159 centre (10, 10) radius 3
  arc A160 (35.9657, 79.8952) -> (44.4663, 82.7551) centre (-0.31, 201.7835) ccw
  arc A161 (-44.9685, 82.7086) -> (-36.9275, 79.8081) centre (2.2046, 200.8918) ccw
  point P0 (-72.5, 87.3979)
  point P1 (-72.5, -87.6021)
  point P2 (72.5, 87.3979)
  point P3 (72.5, -87.6021)
  point P4 (-72.5, 87.3979)
  point P5 (-72.5, -87.6021)
  point P6 (72.5, 87.3979)
  point P7 (72.5, -87.6021)
  point P8 (-72.5, 87.3979)
  point P9 (-72.5, -87.6021)
  point P10 (72.5, 87.3979)
  point P11 (72.5, -87.6021)
  point P12 (-72.5, 87.3979)
  point P13 (-72.5, -87.6021)
  point P14 (72.5, 87.3979)
  point P15 (72.5, -87.6021)
  point P16 (-72.5, 87.3979)
  point P17 (-72.5, -87.6021)
  point P18 (72.5, 87.3979)
  point P19 (72.5, -87.6021)
  point P20 (72.5, -87.6021)
  point P21 (72.5, -87.6021)
  point P22 (72.5, -87.6021)
  point P23 (72.5, -87.6021)
  point P24 (72.5, -87.6021)
sketch "Esboço9" plane through (0, 0, 2) normal (0, 0, 1) x (-1, 0, 0)
sketch "Esboço10" plane through (0, 0, 2) normal (0, 0, 1) x (-1, 0, 0)
  circle A0 centre (-50, 0) radius 2.15
  circle A1 centre (50, 0) radius 2.15
  arc A2 (-89.8492, -89.6213) -> (-86.4551, -92.1669) centre (-86.8794, -89.1971) ccw
  arc A3 (-79.6669, -98.9551) -> (-86.4551, -92.1669) centre (-85.6066, -98.1066) ccw
  arc A4 (-79.6669, -98.9551) -> (-77.1213, -102.3492) centre (-76.6971, -99.3794) ccw
  arc A5 (-77.1213, -102.3492) -> (-73.7447, -102.4474) centre (-75, -87.5) ccw
  arc A6 (-46.7294, -108.889) -> (-73.7447, -102.4474) centre (-70.0264, -146.7235) ccw
  arc A7 (72.6915, -102.3213) -> (44.7852, -108.3244) centre (66.5604, -141.6847) ccw
  arc A8 (72.6915, -102.3213) -> (77.1213, -102.3492) centre (75, -87.5) ccw
  arc A9 (77.1213, -102.3492) -> (79.6669, -98.9551) centre (76.6971, -99.3794) ccw
  arc A10 (86.4551, -92.1669) -> (79.6669, -98.9551) centre (85.6066, -98.1066) ccw
  arc A11 (86.4551, -92.1669) -> (89.8492, -89.6213) centre (86.8794, -89.1971) ccw
  arc A12 (89.8492, -89.6213) -> (89.8492, -85.3787) centre (75, -87.5) ccw
  arc A13 (89.8492, -85.3787) -> (86.4551, -82.8331) centre (86.8794, -85.8029) ccw
  arc A14 (79.7798, -75.4623) -> (86.4551, -82.8331) centre (85.6066, -76.8934) ccw
  arc A15 (79.7798, -75.4623) -> (78.5519, -72.265) centre (76.8663, -74.7468) ccw
  arc A16 (60.7593, -50.7677) -> (78.5519, -72.265) centre (106.6436, -30.9026) ccw
  line L0 (60.7593, -50.7677) -> (52.7268, -32.2145)
  arc A17 (51.9852, -22.4406) -> (52.7268, -32.2145) centre (66.4922, -26.2549) ccw
  arc A18 (51.9852, -22.4406) -> (52.0095, 23.4499) centre (-35.4576, 0.5509) ccw
  arc A19 (52.8518, 33.4268) -> (52.0095, 23.4499) centre (66.5205, 27.2489) ccw
  line L1 (52.8518, 33.4268) -> (60.9948, 51.443)
  arc A20 (78.5458, 72.2669) -> (60.9948, 51.443) centre (106.557, 30.8499) ccw
  arc A21 (78.5458, 72.2669) -> (79.7789, 75.4657) centre (76.8651, 74.7519) ccw
  arc A22 (86.4551, 82.8331) -> (79.7789, 75.4657) centre (85.6066, 76.8934) ccw
  arc A23 (86.4551, 82.8331) -> (89.8492, 85.3787) centre (86.8794, 85.8029) ccw
  arc A24 (89.8492, 85.3787) -> (89.8492, 89.6213) centre (75, 87.5) ccw
  arc A25 (89.8492, 89.6213) -> (86.4551, 92.1669) centre (86.8794, 89.1971) ccw
  arc A26 (79.6669, 98.9551) -> (86.4551, 92.1669) centre (85.6066, 98.1066) ccw
  arc A27 (79.6669, 98.9551) -> (77.1213, 102.3492) centre (76.6971, 99.3794) ccw
  arc A28 (77.1213, 102.3492) -> (72.8787, 102.3492) centre (75, 87.5) ccw
  arc A29 (72.8787, 102.3492) -> (70.3331, 98.9551) centre (73.3029, 99.3794) ccw
  arc A30 (62.5456, 92.3982) -> (70.3331, 98.9551) centre (64.3934, 98.1066) ccw
  arc A31 (62.5456, 92.3982) -> (59.6541, 91.8087) centre (61.6216, 89.544) ccw
  arc A32 (44.4663, 82.7551) -> (59.6541, 91.8087) centre (26.8616, 129.5533) ccw
  line L2 (35.9657, 79.8952) -> (2.1827, 93.0889)
  arc A33 (2.1827, 93.0889) -> (-2.1423, 93.1045) centre (0, 87.5) ccw
  line L3 (-2.1423, 93.1045) -> (-36.9275, 79.8081)
  arc A34 (-59.6538, 91.7779) -> (-44.9685, 82.7086) centre (-26.4329, 129.146) ccw
  arc A35 (-59.6538, 91.7779) -> (-62.5625, 92.3928) centre (-61.6471, 89.5359) ccw
  arc A36 (-70.3331, 98.9551) -> (-62.5625, 92.3928) centre (-64.3934, 98.1066) ccw
  arc A37 (-70.3331, 98.9551) -> (-72.8787, 102.3492) centre (-73.3029, 99.3794) ccw
  arc A38 (-72.8787, 102.3492) -> (-77.1213, 102.3492) centre (-75, 87.5) ccw
  arc A39 (-77.1213, 102.3492) -> (-79.6669, 98.9551) centre (-76.6971, 99.3794) ccw
  arc A40 (-86.4551, 92.1669) -> (-79.6669, 98.9551) centre (-85.6066, 98.1066) ccw
  arc A41 (-86.4551, 92.1669) -> (-89.8492, 89.6213) centre (-86.8794, 89.1971) ccw
  arc A42 (-89.8492, 89.6213) -> (-89.8492, 85.3787) centre (-75, 87.5) ccw
  arc A43 (-89.8492, 85.3787) -> (-86.4551, 82.8331) centre (-86.8794, 85.8029) ccw
  arc A44 (-79.7789, 75.4657) -> (-86.4551, 82.8331) centre (-85.6066, 76.8934) ccw
  arc A45 (-79.7789, 75.4657) -> (-78.5458, 72.2669) centre (-76.8651, 74.7519) ccw
  arc A46 (-60.9948, 51.443) -> (-78.5458, 72.2669) centre (-106.557, 30.8499) ccw
  line L4 (-60.9948, 51.443) -> (-52.8518, 33.4268)
  arc A47 (-52.0095, 23.4499) -> (-52.8518, 33.4268) centre (-66.5205, 27.2489) ccw
  arc A48 (-52.0095, 23.4499) -> (-51.9852, -22.4406) centre (35.4576, 0.5509) ccw
  arc A49 (-52.7268, -32.2145) -> (-51.9852, -22.4406) centre (-66.4922, -26.2549) ccw
  line L5 (-52.7268, -32.2145) -> (-60.7593, -50.7677)
  arc A50 (-78.5519, -72.265) -> (-60.7593, -50.7677) centre (-106.6436, -30.9026) ccw
  arc A51 (-78.5519, -72.265) -> (-79.7798, -75.4623) centre (-76.8663, -74.7468) ccw
  arc A52 (-86.4551, -82.8331) -> (-79.7798, -75.4623) centre (-85.6066, -76.8934) ccw
  arc A53 (-86.4551, -82.8331) -> (-89.8492, -85.3787) centre (-86.8794, -85.8029) ccw
  arc A54 (-89.8492, -85.3787) -> (-89.8492, -89.6213) centre (-75, -87.5) ccw
  circle A55 centre (72.5, -95.6021) radius 1.5
  circle A56 centre (-83, -87.5005) radius 1.5
  circle A57 centre (-75.0002, 95.5) radius 1.5
  circle A58 centre (-67, 87.5002) radius 1.5
  circle A59 centre (83, 87.5) radius 1.5
  circle A60 centre (75, 79.5) radius 1.5
  circle A61 centre (-75, 87.5) radius 3
  circle A62 centre (-74.9995, -95.5) radius 1.5
  circle A63 centre (-75.0005, -79.5) radius 1.5
  circle A64 centre (64.5, -87.6021) radius 1.5
  circle A65 centre (80.5, -87.6021) radius 1.5
  circle A66 centre (-75, -87.5) radius 3
  circle A67 centre (-83, 87.4998) radius 1.5
  circle A68 centre (75, 95.5) radius 1.5
  circle A69 centre (75, 87.5) radius 3
  circle A70 centre (67, 87.5) radius 1.5
  circle A71 centre (-74.9998, 79.5) radius 1.5
  circle A72 centre (-67, -87.4995) radius 1.5
  circle A73 centre (75, -87.5) radius 3
  circle A74 centre (72.5, -79.6021) radius 1.5
  arc A75 (-10.473, -56.6595) -> (-14.3032, -58.4456) centre (-10.473, -61.6595) ccw
  line L6 (-10.473, -56.6595) -> (-7, -56.6595)
  arc A76 (-5, -58.6595) -> (-7, -56.6595) centre (-7, -58.6595) ccw
  line L7 (-5, -58.6595) -> (-5, -97.464)
  arc A77 (-9.1318, -102.3881) -> (-5, -97.464) centre (-10, -97.464) ccw
  line L8 (-9.1318, -102.3881) -> (-26.9725, -105.5339)
  arc A78 (-32.7648, -101.4781) -> (-26.9725, -105.5339) centre (-27.8408, -100.6098) ccw
  line L9 (-32.7648, -101.4781) -> (-35.4243, -86.3954)
  arc A79 (-34.3305, -82.3132) -> (-35.4243, -86.3954) centre (-30.5003, -85.5271) ccw
  line L10 (-34.3305, -82.3132) -> (-14.3032, -58.4456)
  line L11 (6.3787, -9) -> (-6.3787, -9)
  arc A80 (-6.7322, -8.1464) -> (-6.3787, -9) centre (-6.3787, -8.5) ccw
  line L12 (-6.7322, -8.1464) -> (-0.7071, -2.1213)
  arc A81 (0.7071, -2.1213) -> (-0.7071, -2.1213) centre (0, -2.8284) ccw
  line L13 (0.7071, -2.1213) -> (6.7322, -8.1464)
  arc A82 (6.3787, -9) -> (6.7322, -8.1464) centre (6.3787, -8.5) ccw
  arc A83 (8.1464, -6.7322) -> (9, -6.3787) centre (8.5, -6.3787) ccw
  line L14 (8.1464, -6.7322) -> (2.1213, -0.7071)
  arc A84 (2.1213, 0.7071) -> (2.1213, -0.7071) centre (2.8284, 0) ccw
  line L15 (2.1213, 0.7071) -> (8.1464, 6.7322)
  arc A85 (9, 6.3787) -> (8.1464, 6.7322) centre (8.5, 6.3787) ccw
  line L16 (9, 6.3787) -> (9, -6.3787)
  line L17 (5, -97.464) -> (5, -58.6595)
  arc A86 (7, -56.6595) -> (5, -58.6595) centre (7, -58.6595) ccw
  line L18 (7, -56.6595) -> (10.473, -56.6595)
  arc A87 (14.3032, -58.4456) -> (10.473, -56.6595) centre (10.473, -61.6595) ccw
  line L19 (14.3032, -58.4456) -> (34.3305, -82.3132)
  arc A88 (35.4243, -86.3954) -> (34.3305, -82.3132) centre (30.5003, -85.5271) ccw
  line L20 (35.4243, -86.3954) -> (32.7648, -101.4781)
  arc A89 (26.9725, -105.5339) -> (32.7648, -101.4781) centre (27.8408, -100.6098) ccw
  line L21 (26.9725, -105.5339) -> (9.1318, -102.3881)
  arc A90 (5, -97.464) -> (9.1318, -102.3881) centre (10, -97.464) ccw
  arc A91 (38.1376, -9.2791) -> (38.7256, -7.6527) centre (36.7356, -7.8528) ccw
  line L22 (38.1376, -9.2791) -> (27.9736, -19.2699)
  arc A92 (24.5716, -17.8424) -> (27.9736, -19.2699) centre (26.5716, -17.8436) ccw
  line L23 (24.5716, -17.8424) -> (24.5916, 17.8264)
  arc A93 (27.9955, 19.2498) -> (24.5916, 17.8264) centre (26.5916, 17.8253) ccw
  line L24 (27.9955, 19.2498) -> (38.1463, 9.2454)
  arc A94 (38.7321, 7.6192) -> (38.1463, 9.2454) centre (36.7424, 7.821) ccw
  arc A95 (38.7321, 7.6192) -> (38.7256, -7.6527) centre (114.3432, -0.0492) ccw
  arc A96 (-38.7303, -7.6383) -> (-38.142, -9.266) centre (-36.7404, -7.8393) ccw
  arc A97 (-38.7303, -7.6383) -> (-38.7376, 7.7103) centre (-114.3455, 0) ccw
  arc A98 (-38.1438, 9.3455) -> (-38.7376, 7.7103) centre (-36.7479, 7.9132) ccw
  line L25 (-38.1438, 9.3455) -> (-27.9241, 19.3052)
  arc A99 (-24.5283, 17.871) -> (-27.9241, 19.3052) centre (-26.5283, 17.8728) ccw
  line L26 (-24.5283, 17.871) -> (-24.5606, -17.8415)
  arc A100 (-27.9622, -19.2664) -> (-24.5607, -17.8415) centre (-26.5606, -17.8397) ccw
  line L27 (-27.9622, -19.2664) -> (-38.142, -9.266)
  arc A101 (-61.9967, -63.6938) -> (-55.4143, -68.0759) centre (-58.3695, -65.3802) ccw
  line L28 (-61.9967, -63.6938) -> (-41.8922, -17.2564)
  arc A102 (-36.246, -16.5772) -> (-41.8922, -17.2564) centre (-38.8636, -18.6251) ccw
  line L29 (-36.246, -16.5772) -> (-23.6374, -29.1331)
  arc A103 (-23.5625, -33.2372) -> (-23.6374, -29.1331) centre (-25.7596, -31.2246) ccw
  line L30 (-23.5625, -33.2372) -> (-55.4143, -68.0759)
  line L31 (19.3052, -27.9241) -> (9.3455, -38.1438)
  arc A104 (7.7103, -38.7376) -> (9.3455, -38.1438) centre (7.9132, -36.7479) ccw
  arc A105 (7.7103, -38.7376) -> (-7.6383, -38.7303) centre (0, -114.3455) ccw
  arc A106 (-9.266, -38.142) -> (-7.6383, -38.7303) centre (-7.8393, -36.7404) ccw
  line L32 (-9.266, -38.142) -> (-19.2664, -27.9622)
  arc A107 (-17.8415, -24.5606) -> (-19.2664, -27.9622) centre (-17.8397, -26.5606) ccw
  line L33 (-17.8415, -24.5606) -> (17.871, -24.5283)
  arc A108 (19.3052, -27.9241) -> (17.871, -24.5283) centre (17.8728, -26.5283) ccw
  arc A109 (-40.9054, 16.7074) -> (-37.3489, 15.6517) centre (-38.8619, 17.0732) ccw
  line L34 (-40.9054, 16.7074) -> (-46.7322, 29.5993)
  arc A110 (-44.339, 36.0244) -> (-46.7322, 29.5993) centre (-42.0339, 31.5075) ccw
  arc A111 (-44.339, 36.0244) -> (-34.6129, 45.4956) centre (-56.2565, 57.9923) ccw
  arc A112 (-28.1234, 47.5076) -> (-34.6129, 45.4956) centre (-30.28, 42.9921) ccw
  line L35 (-28.1234, 47.5076) -> (-14.9942, 41.2515)
  arc A113 (-14.46, 38.0146) -> (-14.9942, 41.2515) centre (-15.8549, 39.4469) ccw
  line L36 (-14.46, 38.0146) -> (-37.3489, 15.6517)
  arc A114 (9.266, 38.142) -> (7.6383, 38.7303) centre (7.8393, 36.7404) ccw
  line L37 (9.266, 38.142) -> (19.2664, 27.9622)
  arc A115 (17.8415, 24.5606) -> (19.2664, 27.9622) centre (17.8397, 26.5606) ccw
  line L38 (17.8415, 24.5606) -> (-17.871, 24.5283)
  arc A116 (-19.3052, 27.9241) -> (-17.871, 24.5283) centre (-17.8728, 26.5283) ccw
  line L39 (-19.3052, 27.9241) -> (-9.3455, 38.1438)
  arc A117 (-7.7103, 38.7376) -> (-9.3455, 38.1438) centre (-7.9132, 36.7479) ccw
  arc A118 (-7.7103, 38.7376) -> (7.6383, 38.7303) centre (0, 114.3455) ccw
  arc A119 (37.4337, 15.5639) -> (40.6601, 16.1647) centre (38.8376, 16.9884) ccw
  line L40 (37.4337, 15.5639) -> (14.6425, 38.0264)
  arc A120 (15.1963, 41.2612) -> (14.6425, 38.0264) centre (16.0464, 39.4508) ccw
  line L41 (15.1963, 41.2612) -> (28.3187, 47.4234)
  arc A121 (34.7856, 45.3775) -> (28.3187, 47.4234) centre (30.444, 42.8975) ccw
  arc A122 (34.7856, 45.3775) -> (44.4886, 35.8486) centre (56.4937, 57.7776) ccw
  arc A123 (46.6438, 29.4035) -> (44.4886, 35.8486) centre (42.0875, 31.4628) ccw
  line L42 (46.6438, 29.4035) -> (40.6601, 16.1647)
  line L43 (41.7895, -17.0192) -> (61.9965, -63.6935)
  arc A124 (55.3948, -68.0303) -> (61.9965, -63.6935) centre (58.3475, -65.3318) ccw
  line L44 (55.3948, -68.0303) -> (23.5953, -33.2362)
  arc A125 (23.7067, -29.0729) -> (23.5953, -33.2362) centre (25.8097, -31.2123) ccw
  line L45 (23.7067, -29.0729) -> (36.9334, -16.0716)
  arc A126 (41.7895, -17.0192) -> (36.9334, -16.0716) centre (39.0364, -18.2111) ccw
  line L46 (-16.4256, 75.2214) -> (0, 81.5)
  line L47 (0, 81.5) -> (15.6612, 75.3836)
  circle A127 centre (0, 87.5) radius 2.15
  line L48 (-9, -6.3787) -> (-9, 6.3787)
  arc A128 (-8.1464, 6.7322) -> (-9, 6.3787) centre (-8.5, 6.3787) ccw
  line L49 (-8.1464, 6.7322) -> (-2.1213, 0.7071)
  arc A129 (-2.1213, -0.7071) -> (-2.1213, 0.7071) centre (-2.8284, 0) ccw
  line L50 (-2.1213, -0.7071) -> (-8.1464, -6.7322)
  arc A130 (-9, -6.3787) -> (-8.1464, -6.7322) centre (-8.5, -6.3787) ccw
  line L51 (-6.3787, 9) -> (6.3787, 9)
  arc A131 (6.7322, 8.1464) -> (6.3787, 9) centre (6.3787, 8.5) ccw
  line L52 (6.7322, 8.1464) -> (0.7071, 2.1213)
  arc A132 (-0.7071, 2.1213) -> (0.7071, 2.1213) centre (0, 2.8284) ccw
  line L53 (-0.7071, 2.1213) -> (-6.7322, 8.1464)
  arc A133 (-6.3787, 9) -> (-6.7322, 8.1464) centre (-6.3787, 8.5) ccw
  circle A134 centre (-40.65, 60) radius 2.15
  line L54 (47.15, 42.4858) -> (47.15, 67.561)
  arc A135 (49.4611, 71.7764) -> (47.15, 67.561) centre (52.15, 67.561) ccw
  line L55 (49.4611, 71.7764) -> (57.5607, 76.943)
  arc A136 (64.8173, 70.6939) -> (57.5607, 76.943) centre (60.2496, 72.7276) ccw
  line L56 (64.8173, 70.6939) -> (51.1653, 40.0309)
  arc A137 (49.5538, 39.7214) -> (51.1653, 40.0309) centre (50.2517, 40.4376) ccw
  line L57 (49.5538, 39.7214) -> (47.4521, 41.7697)
  arc A138 (47.15, 42.4858) -> (47.4521, 41.7697) centre (48.15, 42.4858) ccw
  circle A139 centre (40.65, 60) radius 2.15
  circle A140 centre (-40.65, 50) radius 2.15
  arc A141 (-57.5607, 76.943) -> (-64.8173, 70.6939) centre (-60.2496, 72.7276) ccw
  line L58 (-57.5607, 76.943) -> (-49.4611, 71.7764)
  arc A142 (-47.15, 67.561) -> (-49.4611, 71.7764) centre (-52.15, 67.561) ccw
  line L59 (-47.15, 67.561) -> (-47.15, 42.4858)
  arc A143 (-47.4521, 41.7697) -> (-47.15, 42.4858) centre (-48.15, 42.4858) ccw
  line L60 (-47.4521, 41.7697) -> (-49.5538, 39.7214)
  arc A144 (-51.1653, 40.0309) -> (-49.5538, 39.7214) centre (-50.2517, 40.4376) ccw
  line L61 (-51.1653, 40.0309) -> (-64.8173, 70.6939)
  circle A145 centre (40.65, 50) radius 2.15
  circle A146 centre (-10.25, -46.6) radius 1.5
  line L62 (8, -42.5) -> (8, -50.7)
  line L63 (8, -50.7) -> (-8, -50.7)
  line L64 (-8, -50.7) -> (-8, -42.5)
  line L65 (-8, -42.5) -> (8, -42.5)
  circle A147 centre (10.25, -46.6) radius 1.5
  circle A148 centre (0, -87.5) radius 2.15
  arc A149 (26.2105, 50.915) -> (27.5676, 55.0697) centre (24.9353, 53.6305) ccw
  line L66 (26.2105, 50.915) -> (10.6059, 43.5872)
  arc A150 (9.3307, 43.3027) -> (10.6059, 43.5872) centre (9.3307, 46.3027) ccw
  line L67 (9.3307, 43.3027) -> (-9.3218, 43.3027)
  arc A151 (-10.6123, 43.5944) -> (-9.3218, 43.3027) centre (-9.3218, 46.3027) ccw
  line L68 (-10.6123, 43.5944) -> (-26.8632, 51.3381)
  arc A152 (-28.1945, 55.5044) -> (-26.8632, 51.3381) centre (-25.5727, 54.0463) ccw
  line L69 (-28.1945, 55.5044) -> (-17.9762, 73.8773)
  arc A153 (-16.4256, 75.2214) -> (-17.9762, 73.8773) centre (-15.3544, 72.4192) ccw
  arc A154 (17.2021, 74.0283) -> (15.6612, 75.3836) centre (14.5698, 72.5892) ccw
  line L70 (17.2021, 74.0283) -> (27.5676, 55.0697)
  arc A155 (-46.7294, -108.889) -> (-25.7561, -114.8285) centre (-25.7561, -74.8285) ccw
  line L71 (-25.7561, -114.8285) -> (22.9214, -114.8285)
  arc A156 (22.9214, -114.8285) -> (44.7852, -108.3244) centre (22.9214, -74.8285) ccw
  circle A157 centre (-10, 10) radius 3
  circle A158 centre (10, -10) radius 3
  circle A159 centre (-10, -10) radius 3
  circle A160 centre (10, 10) radius 3
  arc A161 (35.9657, 79.8952) -> (44.4663, 82.7551) centre (-0.31, 201.7835) ccw
  arc A162 (-44.9685, 82.7086) -> (-36.9275, 79.8081) centre (2.2046, 200.8918) ccw
  point P0 (-72.5, 87.3979)
  point P1 (-72.5, -87.6021)
  point P2 (72.5, 87.3979)
  point P3 (72.5, -87.6021)
  point P4 (-72.5, 87.3979)
  point P5 (-72.5, -87.6021)
  point P6 (72.5, 87.3979)
  point P7 (72.5, -87.6021)
  point P8 (-72.5, 87.3979)
  point P9 (-72.5, -87.6021)
  point P10 (72.5, 87.3979)
  point P11 (72.5, -87.6021)
  point P12 (72.5, -87.6021)
  point P13 (72.5, -87.6021)
  point P14 (72.5, -87.6021)
  point P15 (72.5, -87.6021)
  point P16 (72.5, -87.6021)
  dimension "d154" = 4.3
  dimension "d155" = 87.5
  measures "d154" diameter of A148
  measures "d155" distance of origin A148.centre
hole "Furo2" at (0, 87.5, 2) direction (0, 0, -1) diameter 4.3 end through all